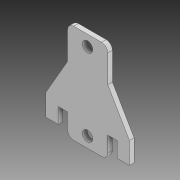
# Autodesk Inventor part: PusherConstraint
Saved by Autodesk Inventor 2020 (Build 240168000, 168)
## iProperties
Created: 2020-11-24
Part Number: PusherConstraint
Material: Generic
Document SubType Name: Modeling
Designer: DDeGo
Density: 1 g/cm^3
Appearance: Default
Author: DDeGo
Autodesk Inventor part; units mm, degrees
ref_plane "YZ Plane" through (0, 0, 0) normal (1, 0, 0) x (0, 1, 0)
ref_plane "XZ Plane" through (0, 0, 0) normal (0, 1, 0) x (-1, 0, 0)
ref_plane "XY Plane" through (0, 0, 0) normal (0, 0, 1) x (1, 0, 0)
sketch "Sketch1" plane through (0, 0, 0) normal (0, 0, 1) x (1, 0, 0)
  line L0 (-6.5, -16) -> (6.5, -16)
  line L1 (6.5, -16) -> (6.5, 16)
  line L2 (6.5, 16) -> (-6.5, 16)
  line L3 (-6.5, 16) -> (-6.5, -16)
  line L4 (-6.5, -16) -> (6.5, 16) construction
  line L5 (6.5, -16) -> (-6.5, 16) construction
  line L6 (0, 0) -> (0, 12.5) construction
  line L7 (0, 0) -> (0, -12.5) construction
  circle A0 centre (0, 12.5) radius 1.65
  circle A1 centre (0, -12.5) radius 1.65
  dimension "d0" = 13
  dimension "d1" = 32
  dimension "d8" = 3.3
  dimension "d9" = 25
  constraints: 16 end point, 2 centre point, 2 coincident, 2 midpoint, 2 parallel, 2 vertical, 1 collinear, 1 equal radius, 1 horizontal, 1 perpendicular
  measures "d0" distance of L1.end L2.end
  measures "d1" distance of L0.end L1.end
  measures "d8" diameter of A0
  measures "d9" distance of L7.end L6.end
extrude "Extrusion1" add sketch "Sketch1" along normal blind 1.5
fillet "Fillet1" radius 2 4 edges at (6.5, 16, 0.75) (-6.5, 16, 0.75) (-6.5, -16, 0.75) (6.5, -16, 0.75)
sketch "Sketch2" plane through (0, 0, 1.5) normal (0, 0, 1) x (1, 0, 0)
  line L0 (6.5, -14) -> (6.5, 14) projected
  line L1 (6.5, -9) -> (9.5, -9)
  line L2 (9.5, -9) -> (9.5, -14)
  line L3 (9.5, -14) -> (6.5, -14) construction
  line L4 (9.5, -14) -> (13.5, -14)
  line L5 (13.5, -14) -> (13.5, -7)
  line L6 (13.5, -7) -> (6.5, 5.1244)
  line L7 (0, 0) -> (0, -8.4482) construction
  line L8 (6.5, 5.1244) -> (6.5, -9)
  line L9 (-6.5, -9) -> (-9.5, -9)
  line L10 (-9.5, -9) -> (-9.5, -14)
  line L11 (-9.5, -14) -> (-6.5, -14) construction
  line L12 (-9.5, -14) -> (-13.5, -14)
  line L13 (-13.5, -14) -> (-13.5, -7)
  line L14 (-13.5, -7) -> (-6.5, 5.1244)
  line L15 (-6.5, 5.1244) -> (-6.5, -9)
  dimension "d10" = 3
  dimension "d11" = 5
  dimension "d12" = 4
  dimension "d13" = 2
  dimension "d14" = 30
  constraints: 30 end point, 7 symmetric about line, 3 perpendicular, 2 horizontal, 2 point on line, 1 collinear, 1 vertical
  measures "d10" distance between parallel lines of L0 L2
  measures "d11" distance of L1.end L2.end
  measures "d12" distance between parallel lines of L5 L2
  measures "d13" distance from line of L5.end L1
  measures "d14" angle of L0 L6
extrude "Extrusion2" add sketch "Sketch2" against normal blind 1.5
body "Solid1"
